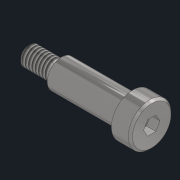
# Autodesk Inventor part: MSB6-15
Saved by Autodesk Inventor 2022.2 (Build 262287010, 287A)
## iProperties
Category: PARTsolutions
Company: MISUMI
Part Number: MSB6-15
Material: 鋼、炭素鋼
Catalog Web Link: www.cadenas.de
Description: MSB, SMSB-Stripper Bolts - Shaft Diameter Tolerance e9
Vendor: MISUMI
Document SubType Name: Modeling
Designer: partserver
Manufacturer: MISUMI
Mass: 5.78001 g
Surface Area: 6.28762 cm^2
Volume: 0.736308 cm^3
Density: 7.85 g/cm^3
Appearance: 半つや出し
PSOL_IDENT_0: {$CADENAS_DATA\23d-libs\misumi\metric\27_screws_nuts\msb.prj},185 {VTYP=3D},{NB=MSB6-15},{LINA=MSB6-
PSOL_IDENT_1: 15},{NN=MSB, SMSB},{DATE=30.06.2021 13:09:33},{GEOMDATE=29.02.2012 02:57:00},{VERSION=},{LINEID=30},
PSOL_IDENT_2: {WBVAR=MAT,ALT1,L,LC,ALT2,FC},{WBNUMERIC=L,LC,FC}  {NB=MSB6-15},{LINA=MSB6-15},{KT=DUMMY},{PN=MSB6-1
PSOL_IDENT_3: 5},{TYPE=MSB},{MAT=},{MAT1= '', '4137 Steel', 'S', '304 Stainless Steel equivalent'  },{HARD=33~38HR
PSOL_IDENT_4: C},{SC=10.9},{D=6.0},{DTOL=-0.020/-0.050},{ALT1=},{ALT1ALG= '','w/o LC (Length (L))','LC','with LC (
PSOL_IDENT_5: Length (L))' },{L=15},{LC=0},{A=9.0},{B=3.0},{C=2.0},{E=4.0},{F=7},{MP=4x0.7},{T=6.5},{LALG=10,15,20
PSOL_IDENT_6: ,25,30,35,40,45,50,55,60,65,70},{M=4.0},{KDM=3.242},{ALT2=},{ALT2ALG= '','Not applicable' },{FC=0.0}
PSOL_IDENT_7: ,{LMIN=10.000},{LMAX=70},{LCALG=0},{FCALG=0},{FCMIN=7.5},{FCMAX=6.5},{FALG=12},{LC1=0.0},{CC=0.300},
PSOL_IDENT_8: {EE=0.700},{S=3.000},{SH=1.200},{P=0.700},{EEE=2.500},{RH=3.261},{RW=0.575},{RR=0.575}
NB: MSB6-15
NN: MSB, SMSB
NT: Stripper Bolts - Shaft Diameter Tolerance e9
NBSYN: $PN.
LINA: MSB6-15
CATALOG: Misumi
PN: MSB6-15
MAT: 4137 Steel
HARD: 33~38HRC
SC: 10.9
D: 6
ALT1: w/o LC (Length (L))
L: 15
LC: 0
A: 9
B: 3
C: 2
E: 4
F: 7
MP: 4x0.7
T: 6.5
ALT2: Not applicable
FC: 0
SUPPLIER: MISUMI
ARTICLENO: MSB6-15
BOMINFO: MSB6-15
CREATOR: CADENAS GmbH
Title: MSB6-15
Author: Cadenas PARTsolutions
Comments: Stripper Bolts - Shaft Diameter Tolerance e9
Autodesk Inventor part; units mm, degrees
ref_plane "YZ Plane" through (0, 0, 0) normal (1, 0, 0) x (0, 1, 0)
ref_plane "XZ Plane" through (0, 0, 0) normal (0, 1, 0) x (-1, 0, 0)
ref_plane "XY Plane" through (0, 0, 0) normal (0, 0, 1) x (1, 0, 0)
sketch "Sketch_7" plane through (0, 0, 0) normal (0, 0, 1) x (1, 0, 0)
  line L0 (22, 0) -> (-1.134, 0)
  line L1 (-1.134, 0) -> (-2, 1.5)
  line L2 (-2, 1.5) -> (-4, 1.5)
  line L3 (-4, 1.5) -> (-4, 4.05)
  line L4 (-4, 4.05) -> (-3.55, 4.5)
  line L5 (-3.55, 4.5) -> (0, 4.5)
  line L6 (0, 4.5) -> (0, 3.25)
  arc A0 (0, 3.25) -> (0.7, 2.7) centre (0.5749, 3.2612) ccw
  line L7 (0.7, 2.7) -> (1, 3)
  line L8 (1, 3) -> (15, 3)
  line L9 (15, 3) -> (15, 1.5)
  line L10 (15, 1.5) -> (15.7, 1.5)
  line L11 (15.7, 1.5) -> (16.2, 2)
  line L12 (16.2, 2) -> (21.5705, 2)
  line L13 (21.5705, 2) -> (22, 1.5705)
  line L14 (22, 1.5705) -> (22, 0)
  line L15 (22, 0) -> (-1.134, 0)
  constraints: 32 end point, 2 point on circle, 1 centre point
revolve "Revolution1" add sketch "Sketch_7" angle 360 about axis through (22, 0, 0) along (1, 0, 0)
thread "Thread1" size "M4x0.7" class "6g" standard "ISO Metric profile" full length
sketch "Sketch_4" plane through (-4, 0, 0) normal (1, 0, 0) x (0, 0, -1)
  line L0 (-1.5, -0.866) -> (0, -1.7321)
  line L1 (0, -1.7321) -> (1.5, -0.866)
  line L2 (1.5, -0.866) -> (1.5, 0.866)
  line L3 (1.5, 0.866) -> (0, 1.7321)
  line L4 (0, 1.7321) -> (-1.5, 0.866)
  line L5 (-1.5, 0.866) -> (-1.5, -0.866)
  constraints: 12 end point
extrude "Extrusion1" cut sketch "Sketch_4" along normal blind 2
body "Solid1"
